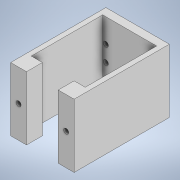
# Autodesk Inventor part: 20220703_Fan Fixed
Saved by Autodesk Inventor 2020 (Build 240168000, 168)
## iProperties
Created: 2022-07-03
Part Number: 20220703_Fan Fixed
Material: 一般
Document SubType Name: Modeling
Designer: Naggy
Density: 1 g/cm^3
Appearance: 既定
Author: Naggy
Autodesk Inventor part; units mm, degrees
ref_plane "YZ Plane" through (0, 0, 0) normal (1, 0, 0) x (0, 1, 0)
ref_plane "XZ Plane" through (0, 0, 0) normal (0, 1, 0) x (-1, 0, 0)
ref_plane "XY Plane" through (0, 0, 0) normal (0, 0, 1) x (1, 0, 0)
sketch "スケッチ1" plane through (0, 0, 0) normal (0, 0, 1) x (1, 0, 0)
  line L0 (-20, -20) -> (20, -20)
  line L1 (20, -20) -> (20, 20)
  line L2 (20, 20) -> (-20, 20)
  line L3 (-20, 20) -> (-20, -20)
  line L4 (-20, -20) -> (20, 20) construction
  line L5 (20, -20) -> (-20, 20) construction
  point P0 (0, 0)
  dimension "d0" = 40
  dimension "d1" = 40
  constraints: 12 end point, 2 midpoint, 2 parallel, 1 horizontal, 1 perpendicular
  measures "d0" distance between parallel lines of L1 L3
  measures "d1" distance between parallel lines of L0 L2
extrude "押し出し1" add sketch "スケッチ1" along normal blind 60
sketch "スケッチ2" plane through (0, 0, 60) normal (0, 0, 1) x (1, 0, 0)
  line L0 (20, 20) -> (-20, 20) projected
  line L1 (10, -20) -> (-10, -20)
  line L2 (-10, -20) -> (-10, 20)
  line L3 (-10, 20) -> (10, 20)
  line L4 (10, 20) -> (10, -20)
  line L5 (10, -20) -> (-10, 20) construction
  line L6 (-10, -20) -> (10, 20) construction
  point P0 (0, 0)
  dimension "d4" = 20
  constraints: 12 end point, 2 midpoint, 2 parallel, 1 horizontal, 1 perpendicular, 1 point on line
  measures "d4" distance between parallel lines of L4 L2
extrude "押し出し2" cut sketch "スケッチ2" against normal blind 55
sketch "スケッチ4" plane through (0, 0, 60) normal (0, 0, 1) x (1, 0, 0)
  point P0 (0, 0)
  point P1 (-15, 0)
  point P2 (15, 0)
  dimension "d7" = 15
  dimension "d8" = 15
  measures "d7" distance of point (-15, 0) point (0, 0)
  measures "d8" distance of point (15, 0) point (0, 0)
hole "穴1" at (-15, 0, 60) at (15, 0, 60) direction (0, 0, -1) diameter 3.2 depth 6 tip angle 118
sketch "スケッチ5" plane through (-20, -20, 0) normal (0, -1, 0) x (1, 0, 0)
  line L0 (0, 60) -> (10, 60) projected
  line L1 (30, 60) -> (40, 60) projected
  line L2 (3, 50) -> (37, 50)
  line L3 (3, 50) -> (3, 5)
  line L4 (3, 5) -> (37, 5)
  line L5 (37, 5) -> (37, 50)
  line L6 (0, 0) -> (0, 60) projected
  line L7 (40, 0) -> (40, 60) projected
  point P0 (20, 0)
  dimension "d16" = 10
  dimension "d17" = 10
  dimension "d20" = 3
  dimension "d21" = 3
  constraints: 8 end point, 2 perpendicular, 1 vertical
  measures "d16" distance from line of L2.start L0
  measures "d17" distance from line of L2.end L1
  measures "d20" distance from line of L6 L2.start
  measures "d21" distance between parallel lines of L7 L5
extrude "押し出し3" cut sketch "スケッチ5" against normal blind 55
sketch "スケッチ7" plane through (0, 0, 0) normal (0, 0, -1) x (-1, 0, 0)
  point P0 (0, 0)
  point P1 (15, -5)
  point P2 (15, 5)
  point P3 (-15, 5)
  point P4 (-15, -5)
  dimension "d37" = 15
  dimension "d38" = 5
  dimension "d39" = 5
  dimension "d40" = 15
  dimension "d41" = 5
  dimension "d42" = 15
  dimension "d43" = 5
  dimension "d44" = 15
  measures "d37" horizontal distance of point (0, 0) point (15, -5)
  measures "d38" vertical distance of point (15, -5) point (0, 0)
  measures "d39" vertical distance of point (0, 0) point (15, 5)
  measures "d40" horizontal distance of point (15, 5) point (0, 0)
  measures "d41" vertical distance of point (-15, 5) point (0, 0)
  measures "d42" horizontal distance of point (-15, 5) point (0, 0)
  measures "d43" vertical distance of point (0, 0) point (-15, -5)
  measures "d44" horizontal distance of point (-15, -5) point (0, 0)
hole "穴3" at (-15, -5, 0) at (-15, 5, 0) at (15, 5, 0) at (15, -5, 0) direction (0, 0, 1) diameter 3.2 depth 8.8 tip angle 118
